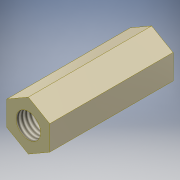
# Autodesk Inventor part: dist25mm
Saved by Autodesk Inventor 2016 (Build 200138000, 138)
## iProperties
Created: 2016-09-22
Part Number: dist25mm
Material: Nylon 6/6
Document SubType Name: Modeling
Designer: Jakub
Density: 1.13 g/cm^3
Appearance: Nylon 6
Mass: 0.460873 g
Surface Area: 7.18248 cm^2
Volume: 0.407853 cm^3
Author: Jakub
Autodesk Inventor part; units mm, degrees
ref_plane "YZ Plane" through (0, 0, 0) normal (1, 0, 0) x (0, 1, 0)
ref_plane "XZ Plane" through (0, 0, 0) normal (0, 1, 0) x (-1, 0, 0)
ref_plane "XY Plane" through (0, 0, 0) normal (0, 0, 1) x (1, 0, 0)
sketch "Sketch1" plane through (0, 0, 0) normal (0, 1, 0) x (-1, 0, 0)
  circle A0 centre (0, 0) radius 1.5
  line L0 (0, -3) -> (-2.5981, -1.5)
  line L1 (-2.5981, -1.5) -> (-2.5981, 1.5)
  line L2 (-2.5981, 1.5) -> (0, 3)
  line L3 (0, 3) -> (2.5981, 1.5)
  line L4 (2.5981, 1.5) -> (2.5981, -1.5)
  line L5 (2.5981, -1.5) -> (0, -3)
  dimension "d0" = 3
  dimension "d1" = 3
  constraints: 12 end point, 2 coincident, 1 centre point, 13 other
  measures "d0" diameter of A0
  measures "d1" distance of L3.end L4.end
extrude "Extrusion1" add sketch "Sketch1" along normal blind 25
thread "Thread1" size "M3x0.5" class "6H" standard "ANSI Metric M Profile" full length
sketch "Sketch2" plane through (0, 0, 0) normal (0, -1, 0) x (1, 0, 0)
  line L0 (-5.778, -4.3605) -> (5.778, -4.3605)
  line L1 (5.778, -4.3605) -> (5.778, 4.3605)
  line L2 (5.778, 4.3605) -> (-5.778, 4.3605)
  line L3 (-5.778, 4.3605) -> (-5.778, -4.3605)
  line L4 (-5.778, -4.3605) -> (5.778, 4.3605) construction
  line L5 (5.778, -4.3605) -> (-5.778, 4.3605) construction
  point P0 (0, 0)
  constraints: 12 end point, 2 midpoint, 2 parallel, 1 horizontal, 1 perpendicular
extrude "Extrusion2" cut sketch "Sketch2" against normal blind 10
body "Solid1"
